Autodesk Inventor part; units mm, degrees
(part 6 of 7)
  line L877 (2.0658, -1.0189) -> (4.0514, -1.0189) projected
  line L878 (-58.6053, 8.1191) -> (-59.4082, 7.5578) projected
  line L879 (-59.4082, 7.5578) -> (-60.7496, 8.4879) projected
  line L880 (-60.7496, 8.4879) -> (-60.7496, 12.7634) projected
  line L881 (-60.7496, 12.7634) -> (-56.4611, 12.7634) projected
  line L882 (-59.4571, 13.4129) -> (-61.4611, 13.4129) projected
  line L883 (-61.4611, 13.4129) -> (-60.7137, 14.7445) projected
  line L884 (-60.7137, 14.7445) -> (-59.6889, 14.7445) projected
  line L885 (-59.6889, 14.7445) -> (-59.3592, 15.0676) projected
  line L886 (-59.3592, 15.0676) -> (-59.3592, 17.2347) projected
  line L887 (-59.3592, 17.2347) -> (-60.743, 17.2347) projected
  line L888 (-60.743, 17.2347) -> (-60.743, 18.5663) projected
  line L889 (-60.743, 18.5663) -> (-56.4611, 18.5663) projected
  line L890 (-56.4611, 18.5663) -> (-56.4611, 14.343) projected
  line L891 (-56.4611, 14.343) -> (-57.8057, 13.4129) projected
  line L892 (-57.8057, 13.4129) -> (-58.762, 14.095) projected
  line L893 (-58.762, 14.095) -> (-59.4571, 13.4129) projected
  line L894 (-56.4611, 29.8554) -> (-56.4611, 24.4344) projected
  line L895 (-56.4611, 24.4344) -> (-57.5218, 25.3515) projected
  line L896 (-57.5218, 25.3515) -> (-57.5218, 26.4807) projected
  line L897 (-57.5218, 26.4807) -> (-60.7137, 26.4807) projected
  line L898 (-60.7137, 26.4807) -> (-61.4611, 27.8123) projected
  line L899 (-61.4611, 27.8123) -> (-57.5218, 27.8123) projected
  line L900 (-57.5218, 27.8123) -> (-57.5218, 28.9416) projected
  line L901 (-57.5218, 28.9416) -> (-56.4611, 29.8554) projected
  line L902 (-75.6403, -50.5982) -> (-75.4415, -50.7741) projected
  line L903 (-75.4415, -50.7741) -> (-75.2314, -50.5982) projected
  line L904 (-75.2314, -50.5982) -> (-75.2314, -48.4484) projected
  line L905 (-75.2314, -48.4484) -> (-74.3267, -47.8041) projected
  line L906 (-74.3267, -47.8041) -> (-73.3854, -48.4689) projected
  line L907 (-73.3854, -48.4689) -> (-73.3854, -51.8113) projected
  line L908 (-73.3854, -51.8113) -> (-74.1279, -51.151) projected
  line L909 (-74.1279, -51.151) -> (-74.1279, -49.0149) projected
  line L910 (-74.1279, -49.0149) -> (-74.3267, -48.8367) projected
  line L911 (-74.3267, -48.8367) -> (-74.5368, -49.0149) projected
  line L912 (-74.5368, -49.0149) -> (-74.5368, -51.1648) projected
  line L913 (-75.6403, -41.3616) -> (-75.6403, -43.7787) projected
  line L914 (-75.6403, -43.7787) -> (-76.3874, -43.1184) projected
  line L915 (-76.3874, -43.1184) -> (-76.3874, -40.4112) projected
  line L916 (-76.3874, -40.4112) -> (-73.4082, -40.4112) projected
  line L917 (-72.8782, -41.3616) -> (-75.6403, -41.3616) projected
  line L918 (-73.3854, -39.4905) -> (-74.3267, -40.1553) projected
  line L919 (-74.3267, -40.1553) -> (-75.4141, -39.3854) projected
  line L920 (-75.4141, -39.3854) -> (-75.4141, -37.4229) projected
  line L921 (-75.4141, -37.4229) -> (-76.8854, -37.4229) projected
  line L922 (-76.8854, -37.4229) -> (-76.3622, -36.4725) projected
  line L923 (-76.3622, -36.4725) -> (-73.3854, -36.4725) projected
  line L924 (-73.3854, -36.4725) -> (-73.3854, -39.4905) projected
  line L925 (-74.5368, -28.9836) -> (-75.4438, -29.6302) projected
  line L926 (-75.4438, -29.6302) -> (-76.3828, -28.9653) projected
  line L927 (-76.3828, -28.9653) -> (-76.3828, -25.623) projected
  line L928 (-76.3828, -25.623) -> (-75.6403, -26.2764) projected
  line L929 (-75.6403, -26.2764) -> (-75.6403, -28.417) projected
  line L930 (-75.6403, -28.417) -> (-75.4415, -28.593) projected
  line L931 (-75.4415, -28.593) -> (-75.2314, -28.417) projected
  line L932 (-75.2314, -28.417) -> (-75.2314, -26.2672) projected
  line L933 (-75.2314, -26.2672) -> (-74.3267, -25.623) projected
  line L934 (-74.3267, -25.623) -> (-73.3854, -26.2878) projected
  line L935 (-73.3854, -26.2878) -> (-73.3854, -29.6302) projected
  line L936 (-73.3854, -29.6302) -> (-74.1279, -28.9699) projected
  line L937 (-74.1279, -28.9699) -> (-74.1279, -26.8338) projected
  line L938 (-74.1279, -26.8338) -> (-74.3267, -26.6556) projected
  line L939 (-74.3267, -26.6556) -> (-74.5368, -26.8338) projected
  line L940 (-74.5368, -26.8338) -> (-74.5368, -28.9836) projected
  line L941 (-75.6403, -19.1804) -> (-75.6403, -21.5975) projected
  line L942 (-75.6403, -21.5975) -> (-76.3874, -20.9373) projected
  line L943 (-76.3874, -20.9373) -> (-76.3874, -18.23) projected
  line L944 (-76.3874, -18.23) -> (-73.4082, -18.23) projected
  line L945 (-73.4082, -18.23) -> (-72.8782, -19.1804) projected
  line L946 (-72.8782, -19.1804) -> (-75.6403, -19.1804) projected
  line L947 (-73.3854, -17.3093) -> (-74.3267, -17.9742) projected
  line L948 (-74.3267, -17.9742) -> (-75.4141, -17.2042) projected
  line L949 (-75.4141, -17.2042) -> (-75.4141, -15.2418) projected
  line L950 (-75.4141, -15.2418) -> (-76.8854, -15.2418) projected
  line L951 (-76.8854, -15.2418) -> (-76.3622, -14.2914) projected
  line L952 (-62.0137, -37.4249) -> (-62.0137, -39.8107) projected
  line L953 (-62.0137, -39.8107) -> (-63.3037, -39.2171) projected
  line L954 (-63.3037, -39.2171) -> (-71.4886, -39.2171) projected
  line L955 (-71.4886, -39.2171) -> (-71.4886, -37.4934) projected
  line L956 (-71.4886, -37.4934) -> (-63.6576, -37.4934) projected
  line L957 (-63.6576, -37.4934) -> (-63.6576, -36.66) projected
  line L958 (-63.6576, -36.66) -> (-62.0137, -37.4249) projected
  line L959 (-69.8448, -24.845) -> (-69.8448, -28.7491) projected
  line L960 (-69.8448, -28.7491) -> (-71.4886, -27.9728) projected
  line L961 (-71.4886, -27.9728) -> (-71.4886, -23.1212) projected
  line L962 (-71.4886, -23.1212) -> (-63.5891, -23.1212) projected
  line L963 (-63.5891, -23.1212) -> (-63.0069, -22.4705) projected
  line L964 (-62.0137, -10.5642) -> (-62.0137, -12.95) projected
  line L965 (-62.0137, -12.95) -> (-63.3037, -12.3564) projected
  line L966 (-63.3037, -12.3564) -> (-71.7398, -12.3564) projected
  line L967 (-71.7398, -12.3564) -> (-64.7078, -7.0938) projected
  line L968 (-64.7078, -7.0938) -> (-69.8448, -7.0938) projected
  line L969 (-69.8448, -7.0938) -> (-69.8448, -9.4911) projected
  line L970 (-69.8448, -9.4911) -> (-71.4886, -8.7263) projected
  line L971 (-71.4886, -8.7263) -> (-71.4886, -5.8381) projected
  line L972 (-71.4886, -5.8381) -> (-70.0731, -6.4888) projected
  line L973 (-70.0731, -6.4888) -> (-63.8973, -6.4888) projected
  line L974 (-63.8973, -6.4888) -> (-63.0069, -5.8381) projected
  line L975 (-63.0069, -5.8381) -> (-61.7398, -7.0596) projected
  line L976 (-61.7398, -7.0596) -> (-68.0297, -11.7514) projected
  line L977 (-68.0297, -11.7514) -> (-63.6576, -11.7514) projected
  line L978 (-63.6576, -11.7514) -> (-63.6576, -9.7993) projected
  line L979 (-63.6576, -9.7993) -> (-62.0137, -10.5642) projected
  line L980 (-64.9704, -4.4454) -> (-69.0571, -4.4454) projected
  line L981 (-70.4727, -5.1075) -> (-71.7398, -3.8861) projected
  line L982 (-69.5252, -2.7331) -> (-66.7284, -2.7331) projected
  line L983 (-66.7284, -2.7331) -> (-66.7284, -0.2445) projected
  line L984 (-66.7284, -0.2445) -> (-71.4886, -0.2445) projected
  line L985 (-71.4886, -0.2445) -> (-71.4886, 1.4792) projected
  line L986 (-71.4886, 1.4792) -> (-63.5891, 1.4792) projected
  line L987 (-63.5891, 1.4792) -> (-63.0069, 2.1299) projected
  line L988 (-66.7284, 12.381) -> (-66.7284, 15.2692) projected
  line L989 (-66.7284, 15.2692) -> (-69.8448, 15.2692) projected
  line L990 (-69.8448, 15.2692) -> (-69.8448, 11.3651) projected
  line L991 (-69.8448, 11.3651) -> (-71.4886, 12.1413) projected
  line L992 (-71.4886, 12.1413) -> (-71.4886, 16.9929) projected
  line L993 (-63.6576, 15.2692) -> (-66.4772, 15.2692) projected
  line L994 (-66.4772, 15.2692) -> (-65.2101, 14.687) projected
  line L995 (-65.2101, 14.687) -> (-65.2101, 11.6733) projected
  line L996 (-65.2101, 11.6733) -> (-66.7284, 12.381) projected
  line L997 (-51.7783, 18.0076) -> (-51.3215, 17.568) projected
  line L998 (-51.3215, 17.568) -> (-50.9232, 17.2377) projected
  line L999 (-50.9232, 17.2377) -> (-50.2693, 16.6848) projected
  line L1000 (-50.2693, 16.6848) -> (-49.9951, 16.4297) projected
  line L1001 (-49.9951, 16.4297) -> (-50.165, 16.3033) projected
  line L1002 (-50.165, 16.3033) -> (-50.5, 16.1442) projected
  line L1003 (-50.5, 16.1442) -> (-51.1005, 15.9331) projected
  line L1004 (-51.1005, 15.9331) -> (-51.8054, 15.7225) projected
  line L1005 (-51.8054, 15.7225) -> (-52.454, 15.5646) projected
  line L1006 (-52.454, 15.5646) -> (-52.9492, 15.4449) projected
  line L1007 (-52.9492, 15.4449) -> (-53.3651, 15.3143) projected
  line L1008 (-53.3651, 15.3143) -> (-53.7749, 15.1819) projected
  line L1009 (-53.7749, 15.1819) -> (-53.8063, 15.279) projected
  line L1010 (-53.8063, 15.279) -> (-53.7947, 15.5136) projected
  line L1011 (-53.7947, 15.5136) -> (-53.3572, 19.0396) projected
  line L1012 (-53.3572, 19.0396) -> (-53.3518, 19.1652) projected
  line L1013 (-53.3518, 19.1652) -> (-53.3854, 19.2823) projected
  line L1014 (-53.3854, 19.2823) -> (-53.6091, 19.5839) projected
  line L1015 (-53.6091, 19.5839) -> (-53.7889, 19.8131) projected
  line L1016 (-53.7889, 19.8131) -> (-53.8265, 19.9093) projected
  line L1017 (-53.8265, 19.9093) -> (-53.8193, 19.9314) projected
  line L1018 (-53.8193, 19.9314) -> (-53.8756, 19.9801) projected
  line L1019 (-53.8756, 19.9801) -> (-53.9256, 20.0367) projected
  line L1020 (-53.9256, 20.0367) -> (-53.8118, 20.0504) projected
  line L1021 (-53.8118, 20.0504) -> (-53.7148, 20.0243) projected
  line L1022 (-53.7148, 20.0243) -> (-53.5909, 19.9446) projected
  line L1023 (-53.5909, 19.9446) -> (-53.2491, 19.6107) projected
  line L1024 (-53.2491, 19.6107) -> (-51.7783, 18.0076) projected
  line L1025 (-50.3026, 20.472) -> (-51.1482, 20.6427) projected
  line L1026 (-51.1482, 20.6427) -> (-52.0028, 20.7487) projected
  line L1027 (-52.0028, 20.7487) -> (-52.9213, 20.8512) projected
  line L1028 (-52.9213, 20.8512) -> (-53.1471, 20.912) projected
  line L1029 (-53.1471, 20.912) -> (-53.2788, 20.9937) projected
  line L1030 (-53.2788, 20.9937) -> (-53.3233, 21.0901) projected
  line L1031 (-53.3233, 21.0901) -> (-53.2667, 21.1656) projected
  line L1032 (-53.2667, 21.1656) -> (-53.1401, 21.2025) projected
  line L1033 (-53.1401, 21.2025) -> (-52.9747, 21.183) projected
  line L1034 (-52.9747, 21.183) -> (-52.2132, 21.067) projected
  line L1035 (-52.2132, 21.067) -> (-51.2901, 20.9848) projected
  line L1036 (-51.2901, 20.9848) -> (-50.8379, 20.9204) projected
  line L1037 (-50.8379, 20.9204) -> (-50.4854, 20.8414) projected
  line L1038 (-50.4854, 20.8414) -> (-49.7014, 20.623) projected
  line L1039 (-49.7014, 20.623) -> (-49.3537, 20.4935) projected
  line L1040 (-49.3537, 20.4935) -> (-49.1396, 20.3844) projected
  line L1041 (-49.1396, 20.3844) -> (-49.029, 20.3131) projected
  line L1042 (-49.029, 20.3131) -> (-48.946, 20.2928) projected
  line L1043 (-48.946, 20.2928) -> (-48.8521, 20.3267) projected
  line L1044 (-48.8521, 20.3267) -> (-48.7091, 20.418) projected
  line L1045 (-48.7091, 20.418) -> (-48.4766, 20.5502) projected
  line L1046 (-48.4766, 20.5502) -> (-48.2708, 20.6349) projected
  line L1047 (-48.2708, 20.6349) -> (-48.1208, 20.6423) projected
  line L1048 (-48.1208, 20.6423) -> (-48.0943, 20.6035) projected
  line L1049 (-48.0943, 20.6035) -> (-48.0878, 20.5284) projected
  line L1050 (-48.0878, 20.5284) -> (-48.1306, 20.4095) projected
  line L1051 (-48.1306, 20.4095) -> (-48.2579, 20.3385) projected
  line L1052 (-48.2579, 20.3385) -> (-48.4307, 20.2573) projected
  line L1053 (-48.4307, 20.2573) -> (-48.6019, 20.108) projected
  line L1054 (-48.6019, 20.108) -> (-48.7427, 19.9228) projected
  line L1055 (-48.7427, 19.9228) -> (-48.8248, 19.734) projected
  line L1056 (-48.8248, 19.734) -> (-48.9463, 19.3465) projected
  line L1057 (-48.9463, 19.3465) -> (-49.0427, 19.0452) projected
  line L1058 (-49.0427, 19.0452) -> (-49.1406, 18.3947) projected
  line L1059 (-49.1406, 18.3947) -> (-49.1671, 17.9451) projected
  line L1060 (-49.1671, 17.9451) -> (-49.1087, 17.5479) projected
  line L1061 (-49.1087, 17.5479) -> (-48.9698, 17.0753) projected
  line L1062 (-48.9698, 17.0753) -> (-48.8063, 16.633) projected
  line L1063 (-48.8063, 16.633) -> (-48.6386, 16.2701) projected
  line L1064 (-48.6386, 16.2701) -> (-48.4868, 16.0355) projected
  line L1065 (-48.4868, 16.0355) -> (-48.3041, 15.8443) projected
  line L1066 (-48.3041, 15.8443) -> (-47.4502, 15.8903) projected
  line L1067 (-47.4502, 15.8903) -> (-46.7506, 15.9386) projected
  line L1068 (-46.7506, 15.9386) -> (-46.2786, 15.9985) projected
  line L1069 (-46.2786, 15.9985) -> (-45.9672, 16.1121) projected
  line L1070 (-45.9672, 16.1121) -> (-45.6158, 16.3115) projected
  line L1071 (-45.6158, 16.3115) -> (-45.2403, 16.5876) projected
  line L1072 (-45.2403, 16.5876) -> (-44.8566, 16.9311) projected
  line L1073 (-44.8566, 16.9311) -> (-44.5098, 17.3449) projected
  line L1074 (-44.5098, 17.3449) -> (-44.1286, 17.9107) projected
  line L1075 (-44.1286, 17.9107) -> (-43.7936, 18.5005) projected
  line L1076 (-43.7936, 18.5005) -> (-43.5854, 18.9863) projected
  line L1077 (-43.5854, 18.9863) -> (-43.4569, 19.3738) projected
  line L1078 (-43.4569, 19.3738) -> (-43.3767, 19.7818) projected
  line L1079 (-43.3767, 19.7818) -> (-43.3327, 20.4387) projected
  line L1080 (-43.3327, 20.4387) -> (-43.3367, 20.7012) projected
  line L1081 (-43.3367, 20.7012) -> (-43.3713, 20.9143) projected
  line L1082 (-43.3713, 20.9143) -> (-43.4509, 21.1367) projected
  line L1083 (-43.4509, 21.1367) -> (-43.5897, 21.4275) projected
  line L1084 (-43.5897, 21.4275) -> (-43.7987, 21.8117) projected
  line L1085 (-43.7987, 21.8117) -> (-43.9901, 22.0986) projected
  line L1086 (-43.9901, 22.0986) -> (-44.1568, 22.2781) projected
  line L1087 (-44.1568, 22.2781) -> (-44.2916, 22.3405) projected
  line L1088 (-44.2916, 22.3405) -> (-44.4801, 22.4154) projected
  line L1089 (-44.4801, 22.4154) -> (-44.8057, 22.5966) projected
  line L1090 (-44.8057, 22.5966) -> (-45.852, 23.1688) projected
  line L1091 (-45.852, 23.1688) -> (-46.8407, 23.6137) projected
  line L1092 (-46.8407, 23.6137) -> (-47.862, 24.0482) projected
  line L1093 (-47.862, 24.0482) -> (-48.7354, 24.4045) projected
  line L1094 (-48.7354, 24.4045) -> (-49.7216, 24.8106) projected
  line L1095 (-49.7216, 24.8106) -> (-50.9261, 25.3244) projected
  line L1096 (-50.9261, 25.3244) -> (-51.358, 25.4849) projected
  line L1097 (-51.358, 25.4849) -> (-51.5813, 25.5448) projected
  line L1098 (-51.5813, 25.5448) -> (-52.0252, 25.6948) projected
  arc A35 (-52.0652, 26.0877) -> (-52.0252, 25.6948) centre (-51.9558, 25.9004) ccw projected
  line L1099 (-52.0652, 26.0877) -> (-51.3968, 25.8193) projected
  line L1100 (-51.3968, 25.8193) -> (-49.9175, 25.2277) projected
  line L1101 (-49.9175, 25.2277) -> (-48.6002, 24.6932) projected
  line L1102 (-48.6002, 24.6932) -> (-47.7937, 24.3584) projected
  line L1103 (-47.7937, 24.3584) -> (-47.1564, 24.0454) projected
  line L1104 (-47.1564, 24.0454) -> (-47.0155, 23.9884) projected
  line L1105 (-47.0155, 23.9884) -> (-46.6961, 23.8893) projected
  line L1106 (-46.6961, 23.8893) -> (-46.252, 23.7057) projected
  line L1107 (-46.252, 23.7057) -> (-45.2196, 23.1839) projected
  line L1108 (-45.2196, 23.1839) -> (-44.3747, 22.736) projected
  line L1109 (-44.3747, 22.736) -> (-44.0527, 22.5468) projected
  line L1110 (-44.0527, 22.5468) -> (-43.7204, 22.2677) projected
  line L1111 (-43.7204, 22.2677) -> (-43.3928, 21.709) projected
  line L1112 (-43.3928, 21.709) -> (-43.0973, 21.0657) projected
  line L1113 (-43.0973, 21.0657) -> (-43.0417, 20.7944) projected
  line L1114 (-43.0417, 20.7944) -> (-43.0222, 20.4472) projected
  line L1115 (-43.0222, 20.4472) -> (-43.0398, 20.0564) projected
  line L1116 (-43.0398, 20.0564) -> (-43.0959, 19.6546) projected
  line L1117 (-43.0959, 19.6546) -> (-43.2066, 19.1823) projected
  line L1118 (-43.2066, 19.1823) -> (-43.3617, 18.6996) projected
  line L1119 (-43.3617, 18.6996) -> (-43.523, 18.3069) projected
  line L1120 (-43.523, 18.3069) -> (-43.6525, 18.1046) projected
  line L1121 (-43.6525, 18.1046) -> (-43.9366, 17.6189) projected
  line L1122 (-43.9366, 17.6189) -> (-44.1239, 17.307) projected
  line L1123 (-44.1239, 17.307) -> (-44.3421, 17.0243) projected
  line L1124 (-44.3421, 17.0243) -> (-44.6358, 16.7208) projected
  line L1125 (-44.6358, 16.7208) -> (-45.0495, 16.3463) projected
  line L1126 (-45.0495, 16.3463) -> (-45.3942, 16.0747) projected
  line L1127 (-45.3942, 16.0747) -> (-45.742, 15.8693) projected
  line L1128 (-45.742, 15.8693) -> (-46.0987, 15.7274) projected
  line L1129 (-46.0987, 15.7274) -> (-46.4705, 15.6464) projected
  line L1130 (-46.4705, 15.6464) -> (-47.0347, 15.6011) projected
  line L1131 (-47.0347, 15.6011) -> (-47.6755, 15.5878) projected
  line L1132 (-47.6755, 15.5878) -> (-48.2288, 15.6059) projected
  line L1133 (-48.2288, 15.6059) -> (-48.5307, 15.6547) projected
  line L1134 (-48.5307, 15.6547) -> (-48.6845, 15.7938) projected
  line L1135 (-48.6845, 15.7938) -> (-48.8538, 16.0229) projected
  line L1136 (-48.8538, 16.0229) -> (-49.1485, 16.652) projected
  line L1137 (-49.1485, 16.652) -> (-49.2499, 16.9453) projected
  line L1138 (-49.2499, 16.9453) -> (-49.2588, 17.0688) projected
  line L1139 (-49.2588, 17.0688) -> (-49.3285, 17.2666) projected
  line L1140 (-49.3285, 17.2666) -> (-49.4065, 17.4636) projected
  line L1141 (-49.4065, 17.4636) -> (-49.4566, 17.6925) projected
  line L1142 (-49.4566, 17.6925) -> (-49.4737, 18.2364) projected
  line L1143 (-49.4737, 18.2364) -> (-49.3806, 18.8791) projected
  line L1144 (-49.3806, 18.8791) -> (-49.1781, 19.6014) projected
  line L1145 (-49.1781, 19.6014) -> (-49.1227, 19.7813) projected
  line L1146 (-49.1227, 19.7813) -> (-49.1099, 19.8939) projected
  line L1147 (-49.1099, 19.8939) -> (-49.1448, 19.9803) projected
  line L1148 (-49.1448, 19.9803) -> (-49.2326, 20.0814) projected
  line L1149 (-49.2326, 20.0814) -> (-49.376, 20.1738) projected
  line L1150 (-49.376, 20.1738) -> (-49.6145, 20.2728) projected
  line L1151 (-49.6145, 20.2728) -> (-50.3026, 20.472) projected
  line L1152 (-45.9525, 18.1279) -> (-45.9298, 18.1594) projected
  line L1153 (-45.9298, 18.1594) -> (-45.8933, 18.1577) projected
  line L1154 (-45.8933, 18.1577) -> (-45.7764, 18.0496) projected
  line L1155 (-45.7764, 18.0496) -> (-45.6289, 17.8868) projected
  line L1156 (-45.6289, 17.8868) -> (-45.7776, 17.7533) projected
  line L1157 (-45.7776, 17.7533) -> (-45.8998, 17.6649) projected
  line L1158 (-45.8998, 17.6649) -> (-46.0012, 17.6307) projected
  line L1159 (-46.0012, 17.6307) -> (-46.0985, 17.6494) projected
  line L1160 (-46.0985, 17.6494) -> (-46.2081, 17.7197) projected
  line L1161 (-46.2081, 17.7197) -> (-46.2717, 17.7714) projected
  line L1162 (-46.2717, 17.7714) -> (-46.2942, 17.8189) projected
  line L1163 (-46.2942, 17.8189) -> (-46.2213, 17.9597) projected
  line L1164 (-46.2213, 17.9597) -> (-46.1283, 18.0616) projected
  line L1165 (-46.1283, 18.0616) -> (-46.0515, 18.079) projected
  line L1166 (-46.0515, 18.079) -> (-45.9994, 18.0796) projected
  line L1167 (-45.9994, 18.0796) -> (-45.9525, 18.1279) projected
  line L1168 (-69.274, 4.3103) -> (-71.7512, 6.2623) projected
  line L1169 (-71.7512, 6.2623) -> (-71.4886, 6.6505) projected
  line L1170 (-71.4886, 6.6505) -> (-71.4886, 8.0888) projected
  line L1171 (-71.4886, 8.0888) -> (-63.5891, 9.9952) projected
  line L1172 (-63.5891, 9.9952) -> (-63.0069, 10.6459) projected
  line L1173 (-64.8334, -16.8769) -> (-64.8334, -19.5368) projected
  line L1174 (-69.0115, -20.7925) -> (-71.7512, -18.6349) projected
  line L1175 (-71.7512, -18.6349) -> (-71.4544, -18.1441) projected
  line L1176 (-69.8448, -32.0253) -> (-69.8448, -35.9409) projected
  line L1177 (-69.8448, -35.9409) -> (-71.4886, -35.1646) projected
  line L1178 (-71.4886, -35.1646) -> (-71.4886, -30.3016) projected
  line L1179 (-71.4886, -30.3016) -> (-63.6576, -30.3016) projected
  line L1180 (-63.6576, -30.3016) -> (-63.6576, -29.4683) projected
  line L1181 (-63.6576, -29.4683) -> (-62.0137, -30.2331) projected
  line L1182 (-71.7512, -45.5299) -> (-71.4658, -45.1418) projected
  line L1183 (-61.7398, -43.0413) -> (-62.0137, -43.4409) projected
  line L1184 (-62.0137, -43.4409) -> (-62.0137, -46.1007) projected
  line L1185 (-62.0137, -46.1007) -> (-62.3905, -45.918) projected
  line L1186 (-64.7078, -50.1874) -> (-69.8448, -50.1874) projected
  line L1187 (-69.8448, -50.1874) -> (-69.8448, -52.5847) projected
  line L1188 (-69.8448, -52.5847) -> (-71.4886, -51.8199) projected
  line L1189 (-71.4886, -51.8199) -> (-71.4886, -48.9317) projected
  line L1190 (-71.4886, -48.9317) -> (-70.0731, -49.5824) projected
  line L1191 (-70.0731, -49.5824) -> (-63.8973, -49.5824) projected
  line L1192 (-63.8973, -49.5824) -> (-63.0069, -48.9317) projected
  line L1193 (-72.8782, -25.1752) -> (-75.6928, -25.1752) projected
  line L1194 (-75.6928, -25.1752) -> (-76.3828, -24.5058) projected
  line L1195 (-76.3828, -24.5058) -> (-76.3828, -22.3309) projected
  line L1196 (-76.3828, -22.3309) -> (-75.6928, -21.6615) projected
  line L1197 (-75.6928, -21.6615) -> (-73.3785, -21.6615) projected
  line L1198 (-73.3785, -21.6615) -> (-73.3854, -22.6119) projected
  line L1199 (-73.3854, -22.6119) -> (-75.6403, -22.6119) projected
  line L1200 (-75.6403, -22.6119) -> (-75.6403, -24.2202) projected
  line L1201 (-75.6403, -24.2202) -> (-73.4082, -24.2202) projected
  line L1202 (-73.4082, -24.2202) -> (-72.8782, -25.1752) projected
  line L1203 (-72.8782, -33.4843) -> (-75.6928, -33.4843) projected
  line L1204 (-75.6928, -33.4843) -> (-76.3828, -32.8149) projected
  line L1205 (-76.3828, -32.8149) -> (-76.3828, -30.6399) projected
  line L1206 (-76.3828, -30.6399) -> (-75.6928, -29.9706) projected
  line L1207 (-75.6928, -29.9706) -> (-73.3785, -29.9706) projected
  line L1208 (-75.6403, -30.921) -> (-75.6403, -32.5293) projected
  line L1209 (-75.6403, -32.5293) -> (-73.4082, -32.5293) projected
  line L1210 (-73.4082, -32.5293) -> (-72.8782, -33.4843) projected
  line L1211 (-72.8782, -47.3563) -> (-75.6928, -47.3563) projected
  line L1212 (-75.6928, -47.3563) -> (-76.3828, -46.6869) projected
  line L1213 (-76.3828, -46.6869) -> (-76.3828, -44.512) projected
  line L1214 (-76.3828, -44.512) -> (-75.6928, -43.8426) projected
  line L1215 (-75.6928, -43.8426) -> (-73.3785, -43.8426) projected
  line L1216 (-73.3785, -43.8426) -> (-73.3854, -44.793) projected
  line L1217 (-73.3854, -44.793) -> (-75.6403, -44.793) projected
  line L1218 (-75.6403, -44.793) -> (-75.6403, -46.4014) projected
  line L1219 (-75.6403, -46.4014) -> (-73.4082, -46.4014) projected
  line L1220 (-73.4082, -46.4014) -> (-72.8782, -47.3563) projected
  line L1221 (-72.8782, -55.6654) -> (-75.6928, -55.6654) projected
  line L1222 (-75.6928, -55.6654) -> (-76.3828, -54.996) projected
  line L1223 (-76.3828, -54.996) -> (-76.3828, -52.8211) projected
  line L1224 (-76.3828, -52.8211) -> (-75.6928, -52.1517) projected
  line L1225 (-75.6928, -52.1517) -> (-73.3785, -52.1517) projected
  line L1226 (-59.7574, 19.1896) -> (-60.743, 20.1263) projected
  line L1227 (-60.743, 20.1263) -> (-60.743, 23.1746) projected
  line L1228 (-60.743, 23.1746) -> (-59.7607, 24.108) projected
  line L1229 (-59.7607, 24.108) -> (-56.4513, 24.108) projected
  line L1230 (-56.4513, 24.108) -> (-56.4611, 22.7764) projected
  line L1231 (-56.4611, 22.7764) -> (-59.6823, 22.7764) projected
  line L1232 (-59.6823, 22.7764) -> (-59.6823, 20.5277) projected
  line L1233 (-57.4467, 1.7484) -> (-59.7574, 1.7484) projected
  line L1234 (-59.7574, 1.7484) -> (-60.743, 2.6851) projected
  line L1235 (-60.743, 2.6851) -> (-60.743, 6.0271) projected
  line L1236 (-60.743, 6.0271) -> (-59.7607, 6.9605) projected
  line L1237 (-59.7607, 6.9605) -> (-57.4434, 6.9605) projected
  line L1238 (-57.4434, 6.9605) -> (-56.4611, 6.0271) projected
  line L1239 (-56.4611, 6.0271) -> (-56.4611, 2.6851) projected
  line L1240 (-56.4611, 2.6851) -> (-57.4467, 1.7484) projected
  line L1241 (4.635, -0.6586) -> (2.0619, -0.6586) projected
  line L1242 (2.0619, -0.6586) -> (2.0619, 0.1032) projected
  line L1243 (2.0619, 0.1032) -> (3.0508, 0.1032) projected
  line L1244 (3.0508, 0.1032) -> (3.0508, 1.3525) projected
  line L1245 (3.0508, 1.3525) -> (2.0795, 1.3525) projected
  line L1246 (2.0795, 1.3525) -> (1.635, 2.1143) projected
  line L1247 (4.635, 1.3525) -> (3.6421, 1.3525) projected
  line L1248 (3.6421, 1.3525) -> (3.6421, 0.1032) projected
  line L1249 (3.6421, 0.1032) -> (4.635, 0.1032) projected
  line L1250 (4.635, 0.1032) -> (4.635, -0.6586) projected
  line L1251 (3.225, -8.5091) -> (2.4946, -7.8354) projected
  line L1252 (2.4946, -7.8354) -> (2.0619, -7.8354) projected
  line L1253 (2.0619, -7.8354) -> (2.0658, -7.0737) projected
  line L1254 (2.0658, -7.0737) -> (4.635, -7.0737) projected
  line L1255 (2.7042, -13.7434) -> (2.7042, -15.6644) projected
  line L1256 (2.7042, -15.6644) -> (2.0619, -15.1396) projected
  line L1257 (2.0619, -15.1396) -> (2.0619, -12.9817) projected
  line L1258 (2.0619, -12.9817) -> (4.6134, -12.9817) projected
  line L1259 (4.6134, -12.9817) -> (5.0697, -13.7434) projected
  line L1260 (5.0697, -13.7434) -> (2.7042, -13.7434) projected
  line L1261 (3.3484, -21.5019) -> (2.8667, -21.8211) projected
  line L1262 (2.8667, -21.8211) -> (2.0619, -21.2924) projected
  line L1263 (2.0619, -21.2924) -> (2.0619, -18.8583) projected
  line L1264 (2.0619, -18.8583) -> (4.635, -18.8583) projected
  line L1265 (2.71, -22.7395) -> (2.0736, -22.7395) projected
  line L1266 (2.0736, -22.7395) -> (2.0736, -22.1559) projected
  line L1267 (2.0736, -22.1559) -> (2.71, -22.1559) projected
  line L1268 (2.71, -22.1559) -> (2.71, -22.7395) projected
  line L1269 (2.6572, -30.8857) -> (2.0658, -30.3531) projected
  line L1270 (2.0658, -30.3531) -> (2.0658, -28.4516) projected
  line L1271 (2.0658, -28.4516) -> (2.6572, -27.919) projected
  line L1272 (2.6572, -27.919) -> (4.0436, -27.919) projected
  line L1273 (4.0436, -27.919) -> (4.635, -28.4516) projected
  line L1274 (2.8961, -33.216) -> (2.8961, -31.9882) projected
  line L1275 (2.8961, -31.9882) -> (2.0658, -31.9882) projected
  line L1276 (2.0658, -31.9882) -> (2.0658, -31.2264) projected
  line L1277 (2.0658, -31.2264) -> (4.635, -31.2264) projected
  line L1278 (4.635, -35.0567) -> (4.635, -37.2852) projected
  line L1279 (4.635, -37.2852) -> (3.9927, -36.7643) projected
  line L1280 (3.9927, -36.7643) -> (3.9927, -35.2858) projected
  line L1281 (3.9927, -35.2858) -> (2.7042, -35.2858) projected
  line L1282 (2.7042, -35.2858) -> (2.7042, -36.4451) projected
  line L1283 (2.7042, -36.4451) -> (3.0527, -36.4451) projected
  line L1284 (3.0527, -36.4451) -> (3.0527, -36.0045) projected
  line L1285 (3.0527, -36.0045) -> (3.6441, -35.5267) projected
  line L1286 (3.6441, -35.5267) -> (3.6441, -37.2069) projected
  line L1287 (3.6441, -37.2069) -> (2.6474, -37.2069) projected
  line L1288 (2.6474, -37.2069) -> (2.0619, -36.6821) projected
  line L1289 (2.0619, -36.6821) -> (2.0619, -35.0567) projected
  line L1290 (2.0619, -35.0567) -> (2.6454, -34.5241) projected
  line L1291 (2.6454, -34.5241) -> (4.0416, -34.5241) projected
  line L1292 (4.0416, -34.5241) -> (4.635, -35.0567) projected
  line L1293 (-38.9396, -7.1334) -> (-40.0969, -7.1334) projected
  line L1294 (-40.0969, -7.1334) -> (-40.0969, -5.8792) projected
  line L1295 (-40.0969, -5.8792) -> (-39.1511, -5.8792) projected
  line L1296 (-39.1511, -5.8792) -> (-38.8515, -5.5708) projected
  line L1297 (-38.8515, -5.5708) -> (-38.8515, -3.5117) projected
  line L1298 (-38.8515, -3.5117) -> (-40.0705, -3.5117) projected
  line L1299 (-40.0705, -3.5117) -> (-40.7431, -2.2574) projected
  line L1300 (-40.7431, -2.2574) -> (-36.2431, -2.2574) projected
  line L1301 (-36.2431, -2.2574) -> (-36.2431, -6.2522) projected
  line L1302 (-38.3139, -6.4872) -> (-38.9396, -7.1334) projected
  line L1303 (-39.2128, -12.685) -> (-40.0969, -11.8008) projected
  line L1304 (-40.0969, -11.8008) -> (-40.0969, -8.6373) projected
  line L1305 (-40.0969, -8.6373) -> (-39.2128, -7.7532) projected
  line L1306 (-39.2128, -7.7532) -> (-37.1273, -7.7532) projected
  line L1307 (-38.1729, -17.6638) -> (-38.8955, -18.1954) projected
  line L1308 (-38.8955, -18.1954) -> (-40.1028, -17.3142) projected
  line L1309 (-40.1028, -17.3142) -> (-40.1028, -13.2695) projected
  line L1310 (-40.1028, -13.2695) -> (-36.2431, -13.2695) projected
  line L1311 (-36.2431, -13.2695) -> (-36.2431, -17.3142) projected
  line L1312 (-36.2431, -17.3142) -> (-37.4504, -18.1954) projected
  line L1313 (-37.4504, -18.1954) -> (-38.1729, -17.6638) projected
  line L1314 (-39.1423, -27.3394) -> (-39.1423, -30.5411) projected
  line L1315 (-39.1423, -30.5411) -> (-40.1028, -29.6687) projected
  line L1316 (-40.1028, -29.6687) -> (-40.1028, -26.0851) projected
  line L1317 (-40.1028, -26.0851) -> (-36.2725, -26.0851) projected
  line L1318 (-36.2725, -26.0851) -> (-35.591, -27.3394) projected
  line L1319 (-35.591, -27.3394) -> (-39.1423, -27.3394) projected
  line L1320 (-73.7525, -68.2) -> (-73.0548, -65.2) projected
  line L1321 (-73.0548, -65.2) -> (-72.4543, -65.2) projected
  line L1322 (-72.4543, -65.2) -> (-71.7566, -68.2) projected
  line L1323 (-71.7566, -68.2) -> (-72.2899, -68.2) projected
  line L1324 (-72.2899, -68.2) -> (-72.4219, -67.5297) projected
  line L1325 (-72.4219, -67.5297) -> (-73.0872, -67.5297) projected
  line L1326 (-73.0872, -67.5297) -> (-73.2193, -68.2) projected
  line L1327 (-70.5731, -68.2) -> (-71.3056, -68.2) projected
  line L1328 (-71.3056, -68.2) -> (-71.3056, -65.2) projected
  line L1329 (-71.3056, -65.2) -> (-70.5731, -65.2) projected
  line L1330 (-69.4767, -66.1219) -> (-69.4767, -67.2781) projected
  line L1331 (-67.1694, -68.2) -> (-68.9236, -68.2) projected
  line L1332 (-68.9236, -68.2) -> (-68.9236, -65.2) projected
  line L1333 (-68.9236, -65.2) -> (-67.1694, -65.2) projected
  line L1334 (-67.1694, -65.2) -> (-67.1694, -65.5912) projected
  line L1335 (-67.1694, -65.5912) -> (-68.4028, -65.5912) projected
  line L1336 (-68.4028, -65.5912) -> (-68.4028, -66.4458) projected
  line L1337 (-68.4028, -66.4458) -> (-67.436, -66.4458) projected
  line L1338 (-68.4028, -66.837) -> (-68.4028, -67.8088) projected
  line L1339 (-68.4028, -67.8088) -> (-67.1694, -67.8088) projected
  line L1340 (-67.1694, -67.8088) -> (-67.1694, -68.2) projected
  line L1341 (-61.9269, -68.2) -> (-61.9269, -65.2) projected
  line L1342 (-61.9269, -65.2) -> (-61.3887, -65.2) projected
  line L1343 (-61.3887, -65.2) -> (-60.5864, -67.3553) projected
  line L1344 (-60.6561, -66.401) -> (-60.6561, -65.2) projected
  circle A36 centre (-9.75, -51.55) radius 1.5 projected
  circle A37 centre (3.25, -51.55) radius 1.5 projected
  circle A38 centre (3.25, -45.05) radius 1.5 projected
  circle A39 centre (3.25, 6.65) radius 1.5 projected
  circle A40 centre (3.25, 13.15) radius 1.5 projected
  circle A41 centre (-9.75, 13.15) radius 1.5 projected
  circle A42 centre (-67.4121, -60.2) radius 1.5 projected
  circle A43 centre (-74.1621, -60.2) radius 1.5 projected
  circle A44 centre (-67.4121, 21.8) radius 1.5 projected
  circle A45 centre (-74.1621, 21.8) radius 1.5 projected
  arc A46 (-34.5609, -6.5715) -> (-34.319, -6.1433) centre (-34.819, -6.1433) ccw projected
  line L1345 (-34.319, -6.1433) -> (-34.319, 1.7) projected
  arc A47 (-33.819, 2.2) -> (-34.319, 1.7) centre (-33.819, 1.7) ccw projected
  line L1346 (-33.819, 2.2) -> (-31.9232, 2.2) projected
  arc A48 (-31.9232, 2.2) -> (-31.4585, 2.8843) centre (-31.9232, 2.7) ccw projected
  arc A49 (-23.3621, 2.3219) -> (-31.4585, 2.8843) centre (-27.2755, 4.5435) ccw projected
  arc A50 (-23.3621, 2.3219) -> (-22.9273, 1.575) centre (-22.9273, 2.075) ccw projected
  line L1347 (-22.9273, 1.575) -> (-21.369, 1.575) projected
  arc A51 (-20.869, 1.075) -> (-21.369, 1.575) centre (-21.369, 1.075) ccw projected
  line L1348 (-20.869, 1.075) -> (-20.869, -6) projected
  arc A52 (-20.869, -6) -> (-20.369, -6.5) centre (-20.369, -6) ccw projected
  line L1349 (-20.369, -6.5) -> (-17.8027, -6.5) projected
  line L1350 (-17.8027, -6.5) -> (-17.8027, -31.5) projected
  line L1351 (-17.8027, -31.5) -> (-22.519, -31.5) projected
  arc A53 (-22.519, -31.5) -> (-23.019, -32) centre (-22.519, -32) ccw projected
  line L1352 (-23.019, -32) -> (-23.019, -39.025) projected
  arc A54 (-23.519, -39.525) -> (-23.019, -39.025) centre (-23.519, -39.025) ccw projected
  line L1353 (-23.519, -39.525) -> (-26.644, -39.525) projected
  arc A55 (-26.644, -39.525) -> (-27.144, -40.025) centre (-26.644, -40.025) ccw projected
  line L1354 (-27.144, -40.025) -> (-27.144, -47.7) projected
  line L1355 (-27.144, -47.7) -> (-32.144, -47.7) projected
  line L1356 (-32.144, -47.7) -> (-32.144, -38.225) projected
  line L1357 (-32.144, -38.225) -> (-28.019, -38.225) projected
  arc A56 (-28.019, -38.225) -> (-27.519, -37.725) centre (-28.019, -37.725) ccw projected
  line L1358 (-27.519, -37.725) -> (-27.519, -32) projected
  arc A57 (-27.519, -32) -> (-28.019, -31.5) centre (-28.019, -32) ccw projected
  line L1359 (-28.019, -31.5) -> (-34.8027, -31.5) projected
  line L1360 (-34.8027, -31.5) -> (-34.8027, -6.9997) projected
  arc A58 (-34.5609, -6.5715) -> (-34.8027, -6.9997) centre (-34.3027, -6.9997) ccw projected
  arc A59 (-41.8371, -69.2) -> (-41.3371, -68.7) centre (-41.8371, -68.7) ccw projected
  line L1361 (-41.3371, -68.7) -> (-41.3371, -49.7) projected
  line L1362 (-41.3371, -49.7) -> (-13, -49.7) projected
  line L1363 (-13, -49.7) -> (-13, -55.4) projected
  line L1364 (-13, -55.4) -> (6.3, -55.4) projected
  line L1365 (6.3, -55.4) -> (6.3, 17) projected
  line L1366 (6.3, 17) -> (-13, 17) projected
  line L1367 (-13, 17) -> (-13, 11.3) projected
  line L1368 (-13, 11.3) -> (-41.3371, 11.3) projected
  line L1369 (-41.3371, 11.3) -> (-41.3371, 30.3) projected
  arc A60 (-41.3371, 30.3) -> (-41.8371, 30.8) centre (-41.8371, 30.3) ccw projected
  line L1370 (-41.8371, 30.8) -> (-78.3805, 30.8) projected
  line L1371 (-78.3805, 30.8) -> (-78.3805, -69.2) projected
  line L1372 (-78.3805, -69.2) -> (-41.8371, -69.2) projected
  line L1373 (-56.7398, -38.1) -> (-56.7398, -0.3) projected
  line L1374 (-56.2398, 0.2) -> (-42.0344, 0.2) projected
  line L1375 (-41.5344, -0.3) -> (-41.5344, -38.1) projected
  line L1376 (-42.0344, -38.6) -> (-56.2398, -38.6) projected
  line L1377 (-15.3027, 0.2) -> (-1.0973, 0.2) projected
  line L1378 (-0.5973, -0.3) -> (-0.5973, -38.1) projected
  line L1379 (-1.0973, -38.6) -> (-15.3027, -38.6) projected
  line L1380 (-15.8027, -38.1) -> (-15.8027, -0.3) projected
  arc A61 (-44.4926, 3.775) -> (-43.9933, 4.2482) centre (-44.4926, 4.275) ccw projected
  line L1381 (-44.4926, 3.775) -> (-49.494, 3.775) projected
  arc A62 (-49.994, 4.275) -> (-49.494, 3.775) centre (-49.494, 4.275) ccw projected
  line L1382 (-49.994, 4.275) -> (-49.994, 9.275) projected
  arc A63 (-49.494, 9.775) -> (-49.994, 9.275) centre (-49.494, 9.275) ccw projected
  line L1383 (-49.494, 9.775) -> (-44.494, 9.775) projected
  arc A64 (-43.994, 9.275) -> (-44.494, 9.775) centre (-44.494, 9.275) ccw projected
  line L1384 (-43.994, 9.275) -> (-43.994, 8.1787) projected
  arc A65 (-43.994, 8.1787) -> (-43.494, 7.6787) centre (-43.494, 8.1787) ccw projected
  line L1385 (-43.494, 7.6787) -> (-38.269, 7.6787) projected
  arc A66 (-37.769, 7.1787) -> (-38.269, 7.6787) centre (-38.269, 7.1787) ccw projected
  line L1386 (-37.769, 7.1787) -> (-37.769, 5.2213) projected
  arc A67 (-38.269, 4.7213) -> (-37.769, 5.2213) centre (-38.269, 5.2213) ccw projected
  line L1387 (-38.269, 4.7213) -> (-43.494, 4.7213) projected
  arc A68 (-43.494, 4.7213) -> (-43.9933, 4.2482) centre (-43.494, 4.2213) ccw projected
  line L1388 (-13.5155, 5.8092) -> (-8.3155, 5.8092) projected
  line L1389 (-8.3155, 5.8092) -> (-8.3155, 0.6092) projected
  line L1390 (-8.3155, 0.6092) -> (-13.5155, 0.6092) projected
  line L1391 (-13.5155, 0.6092) -> (-13.5155, 5.8092) projected
  line L1392 (-21.4873, -42.1072) -> (-16.2873, -42.1072) projected
  line L1393 (-16.2873, -42.1072) -> (-16.2873, -47.3072) projected
  line L1394 (-16.2873, -47.3072) -> (-21.4873, -47.3072) projected
  line L1395 (-21.4873, -47.3072) -> (-21.4873, -42.1072) projected
  circle A69 centre (-17.024, 4.925) radius 1 projected
  line L1396 (-44.206, -67.2781) -> (-44.206, -66.1219) projected
  line L1397 (-44.7815, -65.5912) -> (-44.9933, -65.5912) projected
  line L1398 (-44.9933, -65.5912) -> (-44.9933, -67.8088) projected
  line L1399 (-44.9933, -67.8088) -> (-44.7815, -67.8088) projected
  line L1400 (-49.3787, -66.1992) -> (-49.5606, -67.1385) projected
  line L1401 (-49.5606, -67.1385) -> (-49.0548, -67.1385) projected
  line L1402 (-49.0548, -67.1385) -> (-49.2367, -66.1992) projected
  line L1403 (-72.8256, -66.1992) -> (-73.0075, -67.1385) projected
  line L1404 (-73.0075, -67.1385) -> (-72.5016, -67.1385) projected
  line L1405 (-72.5016, -67.1385) -> (-72.6835, -66.1992) projected
  line L1406 (-69.9975, -67.2781) -> (-69.9975, -66.1219) projected
  line L1407 (-70.5731, -65.5912) -> (-70.7849, -65.5912) projected
  line L1408 (-70.7849, -65.5912) -> (-70.7849, -67.8088) projected
  line L1409 (-70.7849, -67.8088) -> (-70.5731, -67.8088) projected
  line L1410 (-53.5847, -67.3628) -> (-53.5847, -66.0372) projected
  line L1411 (-54.4095, -66.0372) -> (-54.4095, -67.3628) projected
  line L1412 (-56.3181, -65.5912) -> (-56.647, -65.5912) projected
  line L1413 (-56.647, -65.5912) -> (-56.647, -66.6377) projected
  line L1414 (-56.647, -66.6377) -> (-56.3181, -66.6377) projected
  line L1415 (-62.5548, -68.2) -> (-64.1968, -68.2) projected
  line L1416 (-63.1129, -65.5912) -> (-63.1129, -67.8088) projected
  line L1417 (-63.1129, -67.8088) -> (-62.5548, -67.8088) projected
  line L1418 (-62.5548, -67.8088) -> (-62.5548, -68.2) projected
  line L1419 (-75.5864, -68.2) -> (-76.0747, -68.2) projected
  line L1420 (-75.5864, -67.5995) -> (-75.5864, -68.2) projected
  line L1421 (4.6408, -15.7095) -> (4.635, -16.4712) projected
  line L1422 (4.635, -16.4712) -> (2.7022, -16.4712) projected
  line L1423 (4.635, -12.8563) -> (3.9927, -12.3354) projected
  line L1424 (3.9927, -12.3354) -> (3.9927, -10.857) projected
  line L1425 (3.9927, -10.857) -> (2.7042, -10.857) projected
  line L1426 (2.7042, -10.857) -> (2.7042, -12.778) projected
  line L1427 (4.635, -4.7199) -> (4.635, -6.9484) projected
  line L1428 (4.635, -6.9484) -> (3.9927, -6.4275) projected
  line L1429 (3.9927, -6.4275) -> (3.9927, -4.949) projected
  line L1430 (3.9927, -4.949) -> (2.7042, -4.949) projected
  line L1431 (4.0416, -4.1873) -> (4.635, -4.7199) projected
  line L1432 (4.0514, -1.0189) -> (4.635, -1.5515) projected
  line L1433 (4.635, -1.5515) -> (4.635, -3.2865) projected
  line L1434 (4.635, -3.2865) -> (4.0514, -3.8191) projected
  line L1435 (-56.4611, 12.7634) -> (-56.4611, 8.4879) projected
  line L1436 (-56.4611, 8.4879) -> (-57.8024, 7.5578) projected
  line L1437 (-57.8024, 7.5578) -> (-58.6053, 8.1191) projected
  line L1438 (-74.5368, -51.1648) -> (-75.4438, -51.8113) projected
  line L1439 (-75.4438, -51.8113) -> (-76.3828, -51.1465) projected
  line L1440 (-76.3828, -51.1465) -> (-76.3828, -47.8041) projected
  line L1441 (-76.3828, -47.8041) -> (-75.6403, -48.4575) projected
  line L1442 (-75.6403, -48.4575) -> (-75.6403, -50.5982) projected
  line L1443 (-73.4082, -40.4112) -> (-72.8782, -41.3616) projected
  line L1444 (-76.3622, -14.2914) -> (-73.3854, -14.2914) projected
  line L1445 (-73.3854, -14.2914) -> (-73.3854, -17.3093) projected
  line L1446 (-66.7284, -27.7331) -> (-66.7284, -24.845) projected
  line L1447 (-66.7284, -24.845) -> (-69.8448, -24.845) projected
  line L1448 (-63.0069, -22.4705) -> (-61.7398, -23.692) projected
  line L1449 (-61.7398, -23.692) -> (-62.7558, -24.845) projected
  line L1450 (-62.7558, -24.845) -> (-62.0137, -25.1874) projected
  line L1451 (-62.0137, -25.1874) -> (-62.0137, -28.7491) projected
  line L1452 (-62.0137, -28.7491) -> (-63.6576, -27.9728) projected
  line L1453 (-63.6576, -27.9728) -> (-63.6576, -24.845) projected
  line L1454 (-63.6576, -24.845) -> (-66.4772, -24.845) projected
  line L1455 (-66.4772, -24.845) -> (-65.2101, -25.4272) projected
  line L1456 (-65.2101, -25.4272) -> (-65.2101, -28.4409) projected
  line L1457 (-65.2101, -28.4409) -> (-66.7284, -27.7331) projected
  line L1458 (-63.0069, 2.1299) -> (-61.7398, 0.9084) projected
  line L1459 (-61.7398, 0.9084) -> (-62.7558, -0.2445) projected
  line L1460 (-62.7558, -0.2445) -> (-61.7398, -0.9066) projected
  line L1461 (-71.4886, 16.9929) -> (-63.5891, 16.9929) projected
  line L1462 (-63.5891, 16.9929) -> (-63.0069, 17.6436) projected
  line L1463 (-63.0069, 17.6436) -> (-61.7398, 16.4221) projected
  line L1464 (-61.7398, 16.4221) -> (-62.7558, 15.2692) projected
  line L1465 (-62.7558, 15.2692) -> (-62.0137, 14.9267) projected
  line L1466 (-62.0137, 14.9267) -> (-62.0137, 11.3651) projected
  line L1467 (-62.0137, 11.3651) -> (-63.6576, 12.1413) projected
  line L1468 (-63.6576, 12.1413) -> (-63.6576, 15.2692) projected
  line L1469 (-62.0137, 6.2623) -> (-62.0137, 4.1847) projected
  line L1470 (-63.0069, 10.6459) -> (-61.7398, 9.4244) projected
  line L1471 (-61.7398, 9.4244) -> (-62.6302, 8.4199) projected
  line L1472 (-62.6302, 8.4199) -> (-69.8448, 6.6961) projected
  line L1473 (-69.8448, 6.6961) -> (-69.8448, 5.4861) projected
  line L1474 (-69.8448, 5.4861) -> (-69.7192, 5.3947) projected
  line L1475 (-63.6576, 5.2578) -> (-63.6576, 7.0386) projected
  line L1476 (-63.6576, 7.0386) -> (-62.0137, 6.2623) projected
  line L1477 (-61.7398, -16.1806) -> (-62.0137, -16.5801) projected
  line L1478 (-62.0137, -16.5801) -> (-62.0137, -20.4386) projected
  line L1479 (-62.0137, -20.4386) -> (-63.6576, -19.6737) projected
  line L1480 (-63.6576, -19.6737) -> (-63.6576, -15.5642) projected
  line L1481 (-69.8334, -19.4112) -> (-69.4567, -19.7194) projected
  line L1482 (-66.3402, -18.9546) -> (-66.3402, -16.1692) projected
  line L1483 (-66.3402, -16.1692) -> (-64.8334, -16.8769) projected
  line L1484 (-63.3037, -32.0253) -> (-69.8448, -32.0253) projected
  line L1485 (-62.0137, -30.2331) -> (-62.0137, -32.619) projected
  line L1486 (-62.0137, -32.619) -> (-63.3037, -32.0253) projected
  line L1487 (-62.0137, -53.6578) -> (-62.0137, -56.0436) projected
  line L1488 (-62.0137, -56.0436) -> (-63.3037, -55.45) projected
  line L1489 (-63.3037, -55.45) -> (-71.7398, -55.45) projected
  line L1490 (-71.7398, -55.45) -> (-64.7078, -50.1874) projected
  line L1491 (-63.0069, -48.9317) -> (-61.7398, -50.1532) projected
  line L1492 (-61.7398, -50.1532) -> (-68.0297, -54.845) projected
  line L1493 (-68.0297, -54.845) -> (-63.6576, -54.845) projected
  line L1494 (-63.6576, -54.845) -> (-63.6576, -52.8929) projected
  line L1495 (-63.6576, -52.8929) -> (-62.0137, -53.6578) projected
  line L1496 (-73.3785, -29.9706) -> (-73.3854, -30.921) projected
  line L1497 (-73.3854, -30.921) -> (-75.6403, -30.921) projected
  line L1498 (-73.3785, -52.1517) -> (-73.3854, -53.1021) projected
  line L1499 (-73.3854, -53.1021) -> (-75.6403, -53.1021) projected
  line L1500 (-75.6403, -53.1021) -> (-75.6403, -54.7104) projected
  line L1501 (-75.6403, -54.7104) -> (-73.4082, -54.7104) projected
  line L1502 (-73.4082, -54.7104) -> (-72.8782, -55.6654) projected
  line L1503 (-55.7365, 19.1896) -> (-59.7574, 19.1896) projected
  line L1504 (-59.6823, 20.5277) -> (-56.4937, 20.5277) projected
  line L1505 (-56.4937, 20.5277) -> (-55.7365, 19.1896) projected
  line L1506 (1.635, 2.1143) -> (4.635, 2.1143) projected
  line L1507 (4.635, 2.1143) -> (4.635, 1.3525) projected
  line L1508 (4.635, -8.9379) -> (4.635, -9.8015) projected
  line L1509 (4.635, -9.8015) -> (3.6891, -8.9477) projected
  line L1510 (3.6891, -8.9477) -> (2.8354, -9.729) projected
  line L1511 (2.8354, -9.729) -> (2.0795, -9.729) projected
  line L1512 (2.0795, -9.729) -> (1.635, -8.9673) projected
  line L1513 (1.635, -8.9673) -> (2.6944, -8.9673) projected
  line L1514 (2.6944, -8.9673) -> (3.225, -8.5091) projected
  line L1515 (4.635, -7.0737) -> (4.635, -7.8354) projected
  line L1516 (4.635, -7.8354) -> (3.417, -7.8354) projected
  line L1517 (3.417, -7.8354) -> (4.635, -8.9379) projected
  line L1518 (4.635, -18.8583) -> (4.635, -21.2924) projected
  line L1519 (4.635, -21.2924) -> (3.8301, -21.8211) projected
  line L1520 (3.8301, -21.8211) -> (3.3484, -21.5019) projected
  line L1521 (4.0436, -30.8857) -> (2.6572, -30.8857) projected
  line L1522 (4.635, -28.4516) -> (4.635, -30.3531) projected
  line L1523 (4.635, -30.3531) -> (4.0436, -30.8857) projected
  line L1524 (2.8354, -34.1599) -> (1.635, -34.1599) projected
  line L1525 (1.635, -34.1599) -> (2.0834, -33.3981) projected
  line L1526 (2.0834, -33.3981) -> (2.6963, -33.3981) projected
  line L1527 (2.6963, -33.3981) -> (2.8961, -33.216) projected
  line L1528 (4.635, -31.2264) -> (4.635, -33.6311) projected
  line L1529 (4.635, -33.6311) -> (3.8282, -34.1599) projected
  line L1530 (3.8282, -34.1599) -> (3.2544, -33.7721) projected
  line L1531 (3.2544, -33.7721) -> (2.8354, -34.1599) projected
  line L1532 (-36.2431, -6.2522) -> (-37.4533, -7.1334) projected
  line L1533 (-37.4533, -7.1334) -> (-38.3139, -6.4872) projected
  line L1534 (-37.1273, -12.685) -> (-39.2128, -12.685) projected
  line L1535 (-37.1273, -7.7532) -> (-36.2431, -8.6373) projected
  line L1536 (-36.2431, -8.6373) -> (-36.2431, -11.8008) projected
  line L1537 (-36.2431, -11.8008) -> (-37.1273, -12.685) projected
  line L1538 (-73.2193, -68.2) -> (-73.7525, -68.2) projected
  line L1539 (-67.436, -66.4458) -> (-67.436, -66.837) projected
  line L1540 (-67.436, -66.837) -> (-68.4028, -66.837) projected
  line L1541 (-61.4061, -68.2) -> (-61.9269, -68.2) projected
  line L1542 (-60.6561, -65.2) -> (-60.1354, -65.2) projected
  line L1543 (-60.1354, -65.2) -> (-60.1354, -68.2) projected
  line L1544 (-60.1354, -68.2) -> (-60.6736, -68.2) projected
  line L1545 (-60.6736, -68.2) -> (-61.4759, -66.0447) projected
  line L1546 (-61.4061, -66.999) -> (-61.4061, -68.2) projected
  line L1547 (-37.2036, -14.5238) -> (-37.7323, -14.5238) projected
  line L1548 (-37.8763, -3.5117) -> (-37.8763, -5.5766) projected
  line L1549 (4.6408, -15.7095) -> (4.635, -16.4712) projected
  line L1550 (4.635, -16.4712) -> (2.7022, -16.4712) projected
  line L1551 (4.635, -12.8563) -> (3.9927, -12.3354) projected
  line L1552 (3.9927, -12.3354) -> (3.9927, -10.857) projected
  line L1553 (3.9927, -10.857) -> (2.7042, -10.857) projected
  line L1554 (2.7042, -10.857) -> (2.7042, -12.778) projected
  line L1555 (4.635, -4.7199) -> (4.635, -6.9484) projected
  line L1556 (4.635, -6.9484) -> (3.9927, -6.4275) projected
  line L1557 (3.9927, -6.4275) -> (3.9927, -4.949) projected
  line L1558 (3.9927, -4.949) -> (2.7042, -4.949) projected
  line L1559 (4.0416, -4.1873) -> (4.635, -4.7199) projected
  line L1560 (4.0514, -1.0189) -> (4.635, -1.5515) projected
  line L1561 (4.635, -1.5515) -> (4.635, -3.2865) projected
  line L1562 (4.635, -3.2865) -> (4.0514, -3.8191) projected
  line L1563 (-56.4611, 12.7634) -> (-56.4611, 8.4879) projected
  line L1564 (-56.4611, 8.4879) -> (-57.8024, 7.5578) projected
  line L1565 (-57.8024, 7.5578) -> (-58.6053, 8.1191) projected
  line L1566 (-74.5368, -51.1648) -> (-75.4438, -51.8113) projected
  line L1567 (-75.4438, -51.8113) -> (-76.3828, -51.1465) projected
  line L1568 (-76.3828, -51.1465) -> (-76.3828, -47.8041) projected
  line L1569 (-76.3828, -47.8041) -> (-75.6403, -48.4575) projected
  line L1570 (-75.6403, -48.4575) -> (-75.6403, -50.5982) projected
  line L1571 (-73.4082, -40.4112) -> (-72.8782, -41.3616) projected
  line L1572 (-76.3622, -14.2914) -> (-73.3854, -14.2914) projected
  line L1573 (-73.3854, -14.2914) -> (-73.3854, -17.3093) projected
  line L1574 (-66.7284, -27.7331) -> (-66.7284, -24.845) projected
  line L1575 (-66.7284, -24.845) -> (-69.8448, -24.845) projected
  line L1576 (-63.0069, -22.4705) -> (-61.7398, -23.692) projected
  line L1577 (-61.7398, -23.692) -> (-62.7558, -24.845) projected
  line L1578 (-62.7558, -24.845) -> (-62.0137, -25.1874) projected
  line L1579 (-62.0137, -25.1874) -> (-62.0137, -28.7491) projected
  line L1580 (-62.0137, -28.7491) -> (-63.6576, -27.9728) projected
  line L1581 (-63.6576, -27.9728) -> (-63.6576, -24.845) projected
  line L1582 (-63.6576, -24.845) -> (-66.4772, -24.845) projected
  line L1583 (-66.4772, -24.845) -> (-65.2101, -25.4272) projected
  line L1584 (-65.2101, -25.4272) -> (-65.2101, -28.4409) projected
  line L1585 (-65.2101, -28.4409) -> (-66.7284, -27.7331) projected
  line L1586 (-63.0069, 2.1299) -> (-61.7398, 0.9084) projected
  line L1587 (-61.7398, 0.9084) -> (-62.7558, -0.2445) projected
  line L1588 (-62.7558, -0.2445) -> (-61.7398, -0.9066) projected
  line L1589 (-71.4886, 16.9929) -> (-63.5891, 16.9929) projected
  line L1590 (-63.5891, 16.9929) -> (-63.0069, 17.6436) projected
  line L1591 (-63.0069, 17.6436) -> (-61.7398, 16.4221) projected
  line L1592 (-61.7398, 16.4221) -> (-62.7558, 15.2692) projected
  line L1593 (-62.7558, 15.2692) -> (-62.0137, 14.9267) projected
  line L1594 (-62.0137, 14.9267) -> (-62.0137, 11.3651) projected
  line L1595 (-62.0137, 11.3651) -> (-63.6576, 12.1413) projected
  line L1596 (-63.6576, 12.1413) -> (-63.6576, 15.2692) projected
  line L1597 (-62.0137, 6.2623) -> (-62.0137, 4.1847) projected
  line L1598 (-63.0069, 10.6459) -> (-61.7398, 9.4244) projected
  line L1599 (-61.7398, 9.4244) -> (-62.6302, 8.4199) projected
  line L1600 (-62.6302, 8.4199) -> (-69.8448, 6.6961) projected
  line L1601 (-69.8448, 6.6961) -> (-69.8448, 5.4861) projected
  line L1602 (-69.8448, 5.4861) -> (-69.7192, 5.3947) projected
  line L1603 (-63.6576, 5.2578) -> (-63.6576, 7.0386) projected
  line L1604 (-63.6576, 7.0386) -> (-62.0137, 6.2623) projected
  line L1605 (-61.7398, -16.1806) -> (-62.0137, -16.5801) projected
  line L1606 (-62.0137, -16.5801) -> (-62.0137, -20.4386) projected
  line L1607 (-62.0137, -20.4386) -> (-63.6576, -19.6737) projected
  line L1608 (-63.6576, -19.6737) -> (-63.6576, -15.5642) projected
  line L1609 (-69.8334, -19.4112) -> (-69.4567, -19.7194) projected
  line L1610 (-66.3402, -18.9546) -> (-66.3402, -16.1692) projected
  line L1611 (-66.3402, -16.1692) -> (-64.8334, -16.8769) projected
  line L1612 (-63.3037, -32.0253) -> (-69.8448, -32.0253) projected
  line L1613 (-62.0137, -30.2331) -> (-62.0137, -32.619) projected
  line L1614 (-62.0137, -32.619) -> (-63.3037, -32.0253) projected
  line L1615 (-62.0137, -53.6578) -> (-62.0137, -56.0436) projected
  line L1616 (-62.0137, -56.0436) -> (-63.3037, -55.45) projected
  line L1617 (-63.3037, -55.45) -> (-71.7398, -55.45) projected
  line L1618 (-71.7398, -55.45) -> (-64.7078, -50.1874) projected
  line L1619 (-63.0069, -48.9317) -> (-61.7398, -50.1532) projected
  line L1620 (-61.7398, -50.1532) -> (-68.0297, -54.845) projected
  line L1621 (-68.0297, -54.845) -> (-63.6576, -54.845) projected
  line L1622 (-63.6576, -54.845) -> (-63.6576, -52.8929) projected
  line L1623 (-63.6576, -52.8929) -> (-62.0137, -53.6578) projected
  line L1624 (-73.3785, -29.9706) -> (-73.3854, -30.921) projected
  line L1625 (-73.3854, -30.921) -> (-75.6403, -30.921) projected
  line L1626 (-73.3785, -52.1517) -> (-73.3854, -53.1021) projected
  line L1627 (-73.3854, -53.1021) -> (-75.6403, -53.1021) projected
  line L1628 (-75.6403, -53.1021) -> (-75.6403, -54.7104) projected
  line L1629 (-75.6403, -54.7104) -> (-73.4082, -54.7104) projected
  line L1630 (-73.4082, -54.7104) -> (-72.8782, -55.6654) projected
  line L1631 (-55.7365, 19.1896) -> (-59.7574, 19.1896) projected
  line L1632 (-59.6823, 20.5277) -> (-56.4937, 20.5277) projected
  line L1633 (-56.4937, 20.5277) -> (-55.7365, 19.1896) projected
  line L1634 (1.635, 2.1143) -> (4.635, 2.1143) projected
  line L1635 (4.635, 2.1143) -> (4.635, 1.3525) projected
  line L1636 (4.635, -8.9379) -> (4.635, -9.8015) projected
  line L1637 (4.635, -9.8015) -> (3.6891, -8.9477) projected
  line L1638 (3.6891, -8.9477) -> (2.8354, -9.729) projected
  line L1639 (2.8354, -9.729) -> (2.0795, -9.729) projected
  line L1640 (2.0795, -9.729) -> (1.635, -8.9673) projected
  line L1641 (1.635, -8.9673) -> (2.6944, -8.9673) projected
  line L1642 (2.6944, -8.9673) -> (3.225, -8.5091) projected
  line L1643 (4.635, -7.0737) -> (4.635, -7.8354) projected
  line L1644 (4.635, -7.8354) -> (3.417, -7.8354) projected
  line L1645 (3.417, -7.8354) -> (4.635, -8.9379) projected
  line L1646 (4.635, -18.8583) -> (4.635, -21.2924) projected
  line L1647 (4.635, -21.2924) -> (3.8301, -21.8211) projected
  line L1648 (3.8301, -21.8211) -> (3.3484, -21.5019) projected
  line L1649 (4.0436, -30.8857) -> (2.6572, -30.8857) projected
  line L1650 (4.635, -28.4516) -> (4.635, -30.3531) projected
  line L1651 (4.635, -30.3531) -> (4.0436, -30.8857) projected
  line L1652 (2.8354, -34.1599) -> (1.635, -34.1599) projected
  line L1653 (1.635, -34.1599) -> (2.0834, -33.3981) projected
  line L1654 (2.0834, -33.3981) -> (2.6963, -33.3981) projected
  line L1655 (2.6963, -33.3981) -> (2.8961, -33.216) projected
  line L1656 (4.635, -31.2264) -> (4.635, -33.6311) projected
  line L1657 (4.635, -33.6311) -> (3.8282, -34.1599) projected
  line L1658 (3.8282, -34.1599) -> (3.2544, -33.7721) projected
  line L1659 (3.2544, -33.7721) -> (2.8354, -34.1599) projected
  line L1660 (-36.2431, -6.2522) -> (-37.4533, -7.1334) projected
  line L1661 (-37.4533, -7.1334) -> (-38.3139, -6.4872) projected
  line L1662 (-37.1273, -12.685) -> (-39.2128, -12.685) projected
  line L1663 (-37.1273, -7.7532) -> (-36.2431, -8.6373) projected
  line L1664 (-36.2431, -8.6373) -> (-36.2431, -11.8008) projected
  line L1665 (-36.2431, -11.8008) -> (-37.1273, -12.685) projected
  arc A70 (-0.5973, -0.3) -> (-1.0973, 0.2) centre (-1.0973, -0.3) ccw projected
  arc A71 (-1.0973, -38.6) -> (-0.5973, -38.1) centre (-1.0973, -38.1) ccw projected
  arc A72 (-15.8027, -38.1) -> (-15.3027, -38.6) centre (-15.3027, -38.1) ccw projected
  arc A73 (-15.3027, 0.2) -> (-15.8027, -0.3) centre (-15.3027, -0.3) ccw projected
  arc A74 (-56.2398, 0.2) -> (-56.7398, -0.3) centre (-56.2398, -0.3) ccw projected
  arc A75 (-41.5344, -0.3) -> (-42.0344, 0.2) centre (-42.0344, -0.3) ccw projected
  arc A76 (-42.0344, -38.6) -> (-41.5344, -38.1) centre (-42.0344, -38.1) ccw projected
  arc A77 (-56.7398, -38.1) -> (-56.2398, -38.6) centre (-56.2398, -38.1) ccw projected
  arc A78 (-0.5973, -0.3) -> (-1.0973, 0.2) centre (-1.0973, -0.3) ccw projected
  arc A79 (-1.0973, -38.6) -> (-0.5973, -38.1) centre (-1.0973, -38.1) ccw projected
  arc A80 (-15.8027, -38.1) -> (-15.3027, -38.6) centre (-15.3027, -38.1) ccw projected
  arc A81 (-15.3027, 0.2) -> (-15.8027, -0.3) centre (-15.3027, -0.3) ccw projected
  arc A82 (-56.2398, 0.2) -> (-56.7398, -0.3) centre (-56.2398, -0.3) ccw projected
  arc A83 (-41.5344, -0.3) -> (-42.0344, 0.2) centre (-42.0344, -0.3) ccw projected
  arc A84 (-42.0344, -38.6) -> (-41.5344, -38.1) centre (-42.0344, -38.1) ccw projected
  arc A85 (-56.7398, -38.1) -> (-56.2398, -38.6) centre (-56.2398, -38.1) ccw projected
  point P0 (0, 0)
  constraints: 76 other